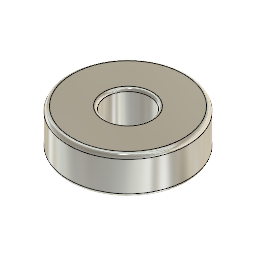
Micro ROV 3 v9 (Autodesk Fusion 360 archive; units mm, degrees)
design "608 Bearing"
Autodesk Fusion 360 part; units mm, degrees
sketch "Sketch1" plane through (0, 0, 0) normal (0, 0, 1) x (1, 0, 0)
  circle A0 centre (0, 0) radius 11
  circle A1 centre (0, 0) radius 4
  dimension "d1" = 22
  dimension "d2" = 8
  measures "d1" diameter of A0
  measures "d2" diameter of A1
extrude "Extrude1" add sketch "Sketch1" along normal blind 7
fillet "Fillet1" radius 0.75 2 edges at (-10.2556, -3.9778, 7) (-10.2556, -3.9778, 0)
fillet "Fillet2" radius 0.5 2 edges at (-3.7293, 1.4465, 7) (-3.7293, 1.4465, 0)
